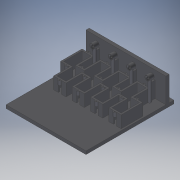
# Autodesk Inventor part: Costas
Saved by Autodesk Inventor 2018 (Build 220112000, 112)
## iProperties
Created: 2017-06-04
Part Number: Costas
Material: Genérico
Document SubType Name: Modeling
Designer: Vitor
Density: 1 g/cm^3
Appearance: Padrão
Author: Vitor
Autodesk Inventor part; units mm, degrees
ref_plane "YZ Plane" through (0, 0, 0) normal (1, 0, 0) x (0, 1, 0)
ref_plane "XZ Plane" through (0, 0, 0) normal (0, 1, 0) x (-1, 0, 0)
ref_plane "XY Plane" through (0, 0, 0) normal (0, 0, 1) x (1, 0, 0)
sketch "Esboço1" plane through (0, 0, 0) normal (0, 0, 1) x (1, 0, 0)
  line L0 (0, 0) -> (100, 0)
  line L1 (100, 0) -> (100, -100)
  line L2 (100, -100) -> (0, -100)
  line L3 (0, -100) -> (0, 0)
  dimension "d0" = 100
  dimension "d1" = 100
  constraints: 8 end point, 2 parallel, 1 horizontal, 1 perpendicular
  measures "d0" distance of L1.end L2.end
  measures "d1" distance of L0.end L1.end
extrude "Extrusão1" add sketch "Esboço1" along normal blind 4
sketch "Esboço2" plane through (0, 0, 4) normal (0, 0, 1) x (1, 0, 0)
  line L0 (100, 0) -> (0, 0) projected
  line L1 (0, 0) -> (4, 0)
  line L2 (4, 0) -> (4, -7)
  line L3 (2, -9) -> (2, -32)
  line L4 (4, -32) -> (4, -9)
  line L5 (2, -32) -> (2, -34)
  line L6 (2, -34) -> (4, -34)
  line L7 (4, -32) -> (15.5, -32)
  line L8 (15.5, -32) -> (15.5, -34)
  line L9 (15.5, -32) -> (13.5, -32)
  line L10 (2, -9) -> (2, -7)
  line L11 (2, -7) -> (4, -7)
  line L12 (15.5, -9) -> (4, -9)
  line L13 (15.5, -7) -> (17.5, -7)
  line L14 (17.5, -7) -> (17.5, -9)
  line L15 (15.5, -9) -> (15.5, -29)
  line L16 (15.5, -29) -> (17.5, -29)
  line L17 (17.5, -27) -> (17.5, -9)
  line L18 (15.5, -29) -> (15.5, -27)
  line L19 (15.5, -29) -> (27, -29)
  line L20 (27, -29) -> (25, -29)
  line L21 (27, -27) -> (27, -29)
  line L22 (25, -27) -> (25, -7)
  line L23 (25, -7) -> (27, -7)
  line L24 (27, -9) -> (27, -27)
  line L25 (15.5, -32) -> (15.5, -52)
  line L26 (15.5, -52) -> (27, -52)
  line L27 (27, -52) -> (27, -32)
  line L28 (13.5, -34) -> (13.5, -52)
  line L29 (13.5, -52) -> (13.5, -54)
  line L30 (13.5, -54) -> (15.5, -54)
  line L31 (27, -54) -> (29, -54)
  line L32 (29, -54) -> (29, -52)
  line L33 (29, -52) -> (29, -34)
  line L34 (29, -32) -> (27, -32)
  line L35 (27, -32) -> (27, -34)
  line L36 (27, -32) -> (38.5, -32)
  line L37 (38.5, -32) -> (36.5, -32)
  line L38 (38.5, -34) -> (38.5, -32)
  line L39 (36.5, -34) -> (36.5, -52)
  line L40 (36.5, -52) -> (36.5, -54)
  line L41 (36.5, -54) -> (38.5, -54)
  line L42 (38.5, -52) -> (38.5, -34)
  line L43 (27, -9) -> (38.5, -9)
  line L44 (38.5, -9) -> (38.5, -27)
  line L45 (38.5, -27) -> (38.5, -29)
  line L46 (38.5, -29) -> (40.5, -29)
  line L47 (40.5, -27) -> (40.5, -9)
  line L48 (40.5, -7) -> (38.5, -7)
  line L49 (40.5, -7) -> (40.5, -9)
  line L50 (38.5, -29) -> (50, -29)
  line L51 (50, -29) -> (50, -27)
  line L52 (50, -52) -> (48, -52)
  line L53 (48, -52) -> (38.5, -52)
  line L54 (50, -34) -> (50, -32)
  line L55 (50, -34) -> (50, -52)
  line L56 (50, -32) -> (52, -32)
  line L57 (52, -34) -> (52, -52)
  line L58 (52, -52) -> (52, -54)
  line L59 (50, -54) -> (52, -54)
  line L60 (50, -32) -> (61.5, -32)
  line L61 (61.5, -32) -> (59.5, -32)
  line L62 (50, -27) -> (50, -9)
  line L63 (50, -7) -> (48, -7)
  line L64 (48, -7) -> (48, -9)
  line L65 (48, -9) -> (48, -27)
  line L66 (50, -9) -> (61.5, -9)
  line L67 (61.5, -7) -> (63.5, -7)
  line L68 (63.5, -7) -> (63.5, -9)
  line L69 (61.5, -9) -> (61.5, -27)
  line L70 (61.5, -27) -> (61.5, -29)
  line L71 (61.5, -29) -> (63.5, -29)
  line L72 (63.5, -27) -> (63.5, -9)
  line L73 (61.5, -34) -> (61.5, -32)
  line L74 (59.5, -34) -> (59.5, -52)
  line L75 (59.5, -52) -> (59.5, -54)
  line L76 (59.5, -54) -> (61.5, -54)
  line L77 (61.5, -52) -> (61.5, -34)
  line L78 (61.5, -52) -> (73, -52)
  line L79 (73, -54) -> (75, -54)
  line L80 (75, -54) -> (75, -52)
  line L81 (73, -52) -> (73, -34)
  line L82 (73, -34) -> (73, -32)
  line L83 (73, -32) -> (75, -32)
  line L84 (75, -34) -> (75, -52)
  line L85 (61.5, -29) -> (73, -29)
  line L86 (73, -29) -> (71, -29)
  line L87 (73, -27) -> (73, -29)
  line L88 (71, -27) -> (71, -9)
  line L89 (71, -9) -> (71, -7)
  line L90 (71, -7) -> (73, -7)
  line L91 (73, -9) -> (73, -27)
  line L92 (73, -9) -> (84.5, -9)
  line L93 (84.5, -7) -> (86.5, -7)
  line L94 (86.5, -7) -> (86.5, -9)
  line L95 (84.5, -9) -> (84.5, -27)
  line L96 (84.5, -27) -> (84.5, -29)
  line L97 (84.5, -29) -> (86.5, -29)
  line L98 (86.5, -27) -> (86.5, -9)
  line L99 (73, -32) -> (84.5, -32)
  line L100 (84.5, -32) -> (84.5, -34)
  line L101 (82.5, -34) -> (82.5, -52)
  line L102 (82.5, -52) -> (82.5, -54)
  line L103 (82.5, -54) -> (84.5, -54)
  line L104 (84.5, -52) -> (84.5, -34)
  line L105 (84.5, -52) -> (96, -52)
  line L106 (96, -54) -> (98, -54)
  line L107 (98, -54) -> (98, -52)
  line L108 (84.5, -29) -> (96, -29)
  line L109 (96, -29) -> (96, -52)
  line L110 (98, -52) -> (98, -29)
  line L111 (98, -29) -> (98, -27)
  line L112 (96, -27) -> (98, -27)
  arc A0 (11.75, -7) -> (7.75, -7) centre (9.75, -7) ccw
  arc A1 (23.25, -27) -> (19.25, -27) centre (21.25, -27) ccw
  arc A2 (19.25, -54) -> (23.25, -54) centre (21.25, -54) ccw
  arc A3 (30.75, -34) -> (34.75, -34) centre (32.75, -34) ccw
  arc A4 (34.75, -7) -> (30.75, -7) centre (32.75, -7) ccw
  arc A5 (46.25, -27) -> (42.25, -27) centre (44.25, -27) ccw
  arc A6 (57.75, -7) -> (53.75, -7) centre (55.75, -7) ccw
  arc A7 (69.25, -27) -> (65.25, -27) centre (67.25, -27) ccw
  arc A8 (80.75, -7) -> (76.75, -7) centre (78.75, -7) ccw
  arc A9 (88.25, -54) -> (92.25, -54) centre (90.25, -54) ccw
  arc A10 (76.75, -34) -> (80.75, -34) centre (78.75, -34) ccw
  arc A11 (65.25, -54) -> (69.25, -54) centre (67.25, -54) ccw
  arc A12 (53.75, -34) -> (57.75, -34) centre (55.75, -34) ccw
  arc A13 (42.25, -54) -> (46.25, -54) centre (44.25, -54) ccw
  line L113 (4, -7) -> (7.75, -7)
  line L114 (11.75, -7) -> (15.5, -7)
  line L115 (27, -7) -> (30.75, -7)
  line L116 (34.75, -7) -> (38.5, -7)
  line L117 (61.5, -7) -> (57.75, -7)
  line L118 (53.75, -7) -> (50, -7)
  line L119 (25, -27) -> (23.25, -27)
  line L120 (19.25, -27) -> (17.5, -27)
  line L121 (84.5, -7) -> (80.75, -7)
  line L122 (76.75, -7) -> (73, -7)
  line L123 (96, -54) -> (92.25, -54)
  line L124 (88.25, -54) -> (84.5, -54)
  line L125 (73, -54) -> (69.25, -54)
  line L126 (65.25, -54) -> (61.5, -54)
  line L127 (38.5, -54) -> (42.25, -54)
  line L128 (46.25, -54) -> (50, -54)
  line L129 (15.5, -54) -> (19.25, -54)
  line L130 (23.25, -54) -> (27, -54)
  line L131 (4, -34) -> (6.75, -34)
  line L132 (11.75, -34) -> (13.5, -34)
  line L133 (36.5, -34) -> (34.75, -34)
  line L134 (30.75, -34) -> (29, -34)
  line L135 (48, -27) -> (46.25, -27)
  line L136 (42.25, -27) -> (40.5, -27)
  line L137 (59.5, -34) -> (57.75, -34)
  line L138 (53.75, -34) -> (52, -34)
  line L139 (63.5, -27) -> (65.25, -27)
  line L140 (69.25, -27) -> (71, -27)
  line L141 (82.5, -34) -> (80.75, -34)
  line L142 (76.75, -34) -> (75, -34)
  line L143 (96, -27) -> (93.25, -27)
  line L144 (88.25, -27) -> (86.5, -27)
  line L145 (92.25, -27) -> (93.25, -27)
  line L146 (6.75, -34) -> (7.75, -34)
  arc A14 (92.25, -27) -> (88.25, -27) centre (90.25, -27) ccw
  arc A15 (7.75, -34) -> (11.75, -34) centre (9.75, -34) ccw
  dimension "d4" = 4
  constraints: 292 end point, 65 point on line, 37 perpendicular, 32 point on circle, 16 centre point, 9 horizontal, 8 vertical, 3 parallel
  measures "d4" distance of L0.end L1.end
extrude "Extrusão3" add sketch "Esboço2" along normal blind 15
sketch "Esboço3" plane through (0, 0, 19) normal (0, 0, 1) x (1, 0, 0)
  line L0 (15.5, -9) -> (4, -9) projected
  line L1 (9.75, -9) -> (9.75, -6.7)
  line L2 (9.75, -6.7) -> (32.75, -6.7)
  line L3 (32.75, -6.7) -> (55.75, -6.7)
  line L4 (55.75, -6.7) -> (78.75, -6.7)
  line L5 (78.75, -6.7) -> (78.75, -34.3)
  line L6 (78.75, -34.3) -> (55.75, -34.3)
  line L7 (55.75, -34.3) -> (32.75, -34.3)
  line L8 (32.75, -34.3) -> (9.75, -34.3)
  line L9 (15.5, -29) -> (27, -29) projected
  line L10 (21.25, -29) -> (21.25, -26.7)
  line L11 (21.25, -26.7) -> (44.25, -26.7)
  line L12 (44.25, -26.7) -> (67.25, -26.7)
  line L13 (67.25, -26.7) -> (90.25, -26.7)
  line L14 (90.25, -26.7) -> (90.25, -54.3)
  line L15 (90.25, -54.3) -> (67.25, -54.3)
  line L16 (88.25, -54) -> (82.5, -54) projected
  line L17 (90.25, -54.3) -> (113.25, -54.3) construction
  line L18 (67.25, -54.3) -> (44.25, -54.3)
  line L19 (44.25, -54.3) -> (21.25, -54.3)
  circle A0 centre (21.25, -54.3) radius 0.75
  circle A1 centre (44.25, -54.3) radius 0.75
  circle A2 centre (67.25, -54.3) radius 0.75
  circle A3 centre (90.25, -54.3) radius 0.75
  circle A4 centre (90.25, -26.7) radius 0.75
  circle A5 centre (78.75, -34.3) radius 0.75
  circle A6 centre (67.25, -26.7) radius 0.75
  circle A7 centre (55.75, -34.3) radius 0.75
  circle A8 centre (44.25, -26.7) radius 0.75
  circle A9 centre (32.75, -34.3) radius 0.75
  circle A10 centre (21.25, -26.7) radius 0.75
  circle A11 centre (9.75, -34.3) radius 0.75
  circle A12 centre (9.75, -6.7) radius 0.75
  circle A13 centre (32.75, -6.7) radius 0.75
  circle A14 centre (55.75, -6.7) radius 0.75
  circle A15 centre (78.75, -6.7) radius 0.75
  point P0 (0, 0)
  dimension "d88" = 2.3
  dimension "d89" = 23
  dimension "d90" = 23
  dimension "d91" = 23
  dimension "d92" = 27.6
  dimension "d93" = 23
  dimension "d94" = 23
  dimension "d95" = 23
  dimension "d96" = 2.3
  dimension "d97" = 23
  dimension "d98" = 23
  dimension "d99" = 23
  dimension "d100" = 27.6
  dimension "d101" = 23
  dimension "d102" = 180
  dimension "d103" = 23
  dimension "d104" = 23
  dimension "d105" = 1.5
  dimension "d106" = 1.5
  dimension "d107" = 1.5
  dimension "d108" = 1.5
  dimension "d109" = 1.5
  dimension "d110" = 1.5
  dimension "d111" = 1.5
  dimension "d112" = 1.5
  dimension "d113" = 1.5
  dimension "d114" = 1.5
  dimension "d115" = 1.5
  dimension "d116" = 1.5
  dimension "d117" = 1.5
  dimension "d118" = 1.5
  dimension "d119" = 1.5
  dimension "d120" = 1.5
  constraints: 34 end point, 16 centre point, 16 coincident, 8 point on line, 5 perpendicular, 2 midpoint, 2 vertical, 1 collinear, 1 horizontal, 1 parallel
  measures "d88" distance of L1.start L1.end
  measures "d89" distance of L1.end L2.end
  measures "d90" distance of L2.end L3.end
  measures "d91" distance of L3.end L4.end
  measures "d92" distance of L4.end L5.end
  measures "d93" distance of L5.end L6.end
  measures "d94" distance of L6.end L7.end
  measures "d95" distance of L7.end L8.end
  measures "d96" distance of L10.start L10.end
  measures "d97" distance of L10.end L11.end
  measures "d98" distance of L11.end L12.end
  measures "d99" distance of L12.end L13.end
  measures "d100" distance of L13.end L14.end
  measures "d101" distance of L14.end L15.end
  measures "d102" angle of L15 L17
  measures "d103" distance of L15.end L18.end
  measures "d104" distance of L18.end L19.end
  measures "d105" diameter of A0
  measures "d106" diameter of A1
  measures "d107" diameter of A2
  measures "d108" diameter of A3
  measures "d109" diameter of A4
  measures "d110" diameter of A5
  measures "d111" diameter of A6
  measures "d112" diameter of A7
  measures "d113" diameter of A8
  measures "d114" diameter of A9
  measures "d115" diameter of A10
  measures "d116" diameter of A11
  measures "d117" diameter of A12
  measures "d118" diameter of A13
  measures "d119" diameter of A14
  measures "d120" diameter of A15
extrude "Extrusão4" cut sketch "Esboço3" against normal blind 10
sketch "Esboço4" plane through (0, 0, 4) normal (0, 0, 1) x (1, 0, 0)
  line L0 (17.5, -7) -> (11.75, -7) projected
  circle A0 centre (17.5, -7) radius 2
  circle A1 centre (40.6139, -7) radius 2
  line L1 (63.5, -27) -> (63.5, -7) projected
  circle A2 centre (63.5, -7) radius 2
  line L2 (86.5, -7) -> (80.75, -7) projected
  circle A3 centre (86.5, -7) radius 2
  point P0 (0, 0)
  dimension "d123" = 4
  dimension "d124" = 4
  dimension "d125" = 4
  dimension "d126" = 4
  constraints: 4 centre point
  measures "d123" diameter of A0
  measures "d124" diameter of A1
  measures "d125" diameter of A2
  measures "d126" diameter of A3
extrude "Extrusão5" add sketch "Esboço4" along normal blind 25
sketch "Esboço5" plane through (86.5, -7, 29) normal (0, 0, 1) x (1, 0, 0)
  line L0 (0, 0) -> (-1, 0)
  line L1 (-1, 0) -> (-1, 1)
  line L2 (-1, 1) -> (1, 1)
  line L3 (1, 1) -> (1, 0)
  line L4 (1, 0) -> (0, 0)
  circle A0 centre (-23, 0) radius 2 projected
  line L5 (-23, 0) -> (-24, 0)
  line L6 (-24, 0) -> (-24, 1)
  line L7 (-24, 1) -> (-22, 1)
  line L8 (-22, 1) -> (-22, 0)
  line L9 (-22, 0) -> (-23, 0)
  arc A1 (-46, -1.9968) -> (-47.8861, 0) centre (-45.8861, 0) ccw projected
  line L10 (-45.8861, 0) -> (-44.8861, 0)
  line L11 (-44.8861, 0) -> (-44.8861, 1)
  line L12 (-44.8861, 1) -> (-46.8861, 1)
  line L13 (-46.8861, 1) -> (-46.8861, 0)
  line L14 (-46.8861, 0) -> (-45.8861, 0)
  circle A2 centre (-69, 0) radius 2 projected
  line L15 (-69, 0) -> (-70, 0)
  line L16 (-70, 0) -> (-70, 1)
  line L17 (-70, 1) -> (-68, 1)
  line L18 (-68, 1) -> (-68, 0)
  line L19 (-68, 0) -> (-69, 0)
  point P0 (-86.5, 7)
  dimension "d129" = 1
  dimension "d130" = 1
  dimension "d131" = 2
  dimension "d132" = 1
  dimension "d133" = 2
  dimension "d134" = 1
  dimension "d135" = 1
  dimension "d136" = 1
  dimension "d137" = 2
  dimension "d138" = 1
  dimension "d139" = 1
  dimension "d140" = 2
  dimension "d141" = 1
  constraints: 40 end point, 11 perpendicular, 10 point on line, 1 horizontal, 1 vertical
  measures "d129" distance of L0.start L0.end
  measures "d130" distance of L0.end L1.end
  measures "d131" distance of L1.end L2.end
  measures "d132" distance of L5.start L5.end
  measures "d133" distance of L6.end L7.end
  measures "d134" distance of L7.end L8.end
  measures "d135" distance of L10.start L10.end
  measures "d136" distance of L10.end L11.end
  measures "d137" distance of L11.end L12.end
  measures "d138" distance of L15.start L15.end
  measures "d139" distance of L15.end L16.end
  measures "d140" distance of L16.end L17.end
  measures "d141" distance of L17.end L18.end
extrude "Extrusão6" add sketch "Esboço5" along normal blind 2 contours L0 L1 L2 L3 L4 | L5 L6 L7 L8 L9 | L14 L13 L12 L11 L10 | L15 L16 L17 L18 L19
sketch "Esboço6" plane through (62.5, -6, 29) normal (0, 1, 0) x (1, 0, 0)
  line L0 (2, -2) -> (0, -2) projected
  circle A0 centre (1, -2) radius 3
  line L1 (25, -2) -> (23, -2) projected
  circle A1 centre (24, -2) radius 3
  line L2 (-22.8861, -2) -> (-20.8861, -2) projected
  circle A2 centre (-21.8861, -2) radius 3
  line L3 (-46, -2) -> (-44, -2) projected
  circle A3 centre (-45, -2) radius 3
  point P0 (-62.5, 29)
  dimension "d144" = 6
  dimension "d145" = 6
  dimension "d146" = 6
  dimension "d147" = 6
  constraints: 4 centre point, 4 midpoint
  measures "d144" diameter of A0
  measures "d145" diameter of A1
  measures "d146" diameter of A2
  measures "d147" diameter of A3
extrude "Extrusão7" add sketch "Esboço6" along normal blind 2 and the other way blind 1
sketch "Esboço7" plane through (61.5, -7, 29) normal (0, -1, 0) x (1, 0, 0)
  circle A0 centre (-44, 2) radius 3 projected
  circle A1 centre (-44, 2) radius 3
  circle A2 centre (-20.8861, 2) radius 3 projected
  circle A3 centre (-20.8861, 2) radius 3
  circle A4 centre (2, 2) radius 3 projected
  circle A5 centre (2, 2) radius 3
  circle A6 centre (25, 2) radius 3 projected
  circle A7 centre (25, 2) radius 3
  point P0 (-61.5, -29)
  dimension "d152" = 6
  dimension "d153" = 6
  dimension "d154" = 6
  dimension "d155" = 6
  constraints: 4 centre point, 4 coincident
  measures "d152" diameter of A1
  measures "d153" diameter of A3
  measures "d154" diameter of A5
  measures "d155" diameter of A7
extrude "Extrusão8" add sketch "Esboço7" along normal blind 3
sketch "Esboço8" plane through (17.5, -10, 31) normal (0, -1, 0) x (1, 0, 0)
  circle A0 centre (0, 0) radius 3 projected
  circle A1 centre (0, 0) radius 1.5
  circle A2 centre (23.1139, 0) radius 3 projected
  circle A3 centre (23.1139, 0) radius 1.5
  circle A4 centre (46, 0) radius 3 projected
  circle A5 centre (46, 0) radius 1.5
  circle A6 centre (69, 0) radius 3 projected
  circle A7 centre (69, 0) radius 1.5
  point P0 (-17.5, -31)
  dimension "d158" = 3
  dimension "d159" = 3
  dimension "d160" = 3
  dimension "d161" = 3
  constraints: 4 centre point, 4 coincident
  measures "d158" diameter of A1
  measures "d159" diameter of A3
  measures "d160" diameter of A5
  measures "d161" diameter of A7
extrude "Extrusão9" cut sketch "Esboço8" against normal blind 7 contours A1 | A3 | A5 | A7
fillet "Arredondamento1" radius 1 8 edges at (39.1139, -10, 31) (62, -10, 31) (85, -10, 31) (16, -10, 31) (85, -4, 31) (62, -4, 31) (39.1139, -4, 31) (16, -4, 31)
sketch "Esboço9" plane through (2, -34, 4) normal (0, -1, 0) x (1, 0, 0)
  line L0 (5.75, 0) -> (5.75, 15) projected
  line L1 (5.75, 0) -> (5.75, 10)
  line L2 (5.75, 10) -> (9.75, 10)
  line L3 (9.75, 0) -> (9.75, 15) projected
  line L4 (9.75, 10) -> (9.75, 0)
  line L5 (9.75, 0) -> (5.75, 0)
  line L6 (2, 0) -> (13.5, 0) projected
  line L7 (28.75, 0) -> (28.75, 15) projected
  line L8 (28.75, 0) -> (28.75, 10)
  line L9 (28.75, 10) -> (32.75, 10)
  line L10 (32.75, 0) -> (32.75, 15) projected
  line L11 (32.75, 0) -> (28.75, 0)
  line L12 (51.75, 0) -> (55.75, 0) projected
  line L13 (51.75, 0) -> (55.75, 0)
  line L14 (28.75, 10) -> (32.75, 10)
  line L15 (51.75, 0) -> (51.75, 10)
  line L16 (51.75, 10) -> (55.75, 10)
  line L17 (55.75, 0) -> (55.75, 15) projected
  line L18 (55.75, 10) -> (55.75, 0)
  line L19 (55.75, 0) -> (51.75, 0)
  line L20 (74.75, 0) -> (74.75, 15) projected
  line L21 (74.75, 0) -> (74.75, 10)
  line L22 (74.75, 10) -> (78.75, 10)
  line L23 (78.75, 0) -> (78.75, 15) projected
  line L24 (78.75, 10) -> (78.75, 0)
  line L25 (98, 0) -> (-2, 0) projected
  line L26 (78.75, 0) -> (74.75, 0)
  line L27 (55.75, 10) -> (51.75, 10)
  line L28 (55.75, 0) -> (51.75, 0)
  line L29 (32.75, 10) -> (28.75, 10)
  line L30 (32.75, 10) -> (32.75, 0)
  line L31 (28.75, 0) -> (32.75, 0) projected
  line L32 (32.75, 0) -> (28.75, 0)
  line L33 (5.75, 10) -> (9.75, 10)
  line L34 (11.5, 0) -> (9.75, 0) projected
  line L35 (5.75, 0) -> (9.75, 0)
  point P0 (-2, -4)
  dimension "d165" = 10
  dimension "d166" = 4
  dimension "d167" = 10
  dimension "d168" = 10
  dimension "d169" = 10
  constraints: 48 end point, 10 collinear, 8 point on line, 3 horizontal, 3 perpendicular, 2 other
  measures "d165" distance of L0.start L1.end
  measures "d166" distance of L1.end L2.end
  measures "d167" distance of L7.start L8.end
  measures "d168" distance of L12.start L15.end
  measures "d169" distance of L20.start L21.end
extrude "Extrusão10" cut sketch "Esboço9" along normal blind 7 and the other way blind 3.5
sketch "Esboço10" plane through (13.5, -54, 4) normal (0, -1, 0) x (1, 0, 0)
  line L0 (5.75, 0) -> (5.75, 15) projected
  line L1 (5.75, 0) -> (5.75, 10)
  line L2 (5.75, 10) -> (9.75, 10)
  line L3 (9.75, 0) -> (9.75, 15) projected
  line L4 (9.75, 0) -> (9.75, 10)
  line L5 (9.75, 0) -> (5.75, 0)
  line L6 (2, 0) -> (13.5, 0) projected
  line L7 (28.75, 0) -> (28.75, 15) projected
  line L8 (28.75, 0) -> (28.75, 10)
  line L9 (28.75, 10) -> (32.75, 10)
  line L10 (32.75, 0) -> (32.75, 15) projected
  line L11 (32.75, 10) -> (32.75, 0)
  line L12 (32.75, 0) -> (28.75, 0)
  line L13 (51.75, 0) -> (51.75, 15) projected
  line L14 (51.75, 0) -> (51.75, 10)
  line L15 (51.75, 10) -> (55.75, 10)
  line L16 (55.75, 0) -> (55.75, 15) projected
  line L17 (55.75, 10) -> (55.75, 0)
  line L18 (55.75, 0) -> (51.75, 0)
  line L19 (48, 0) -> (59.5, 0) projected
  line L20 (74.75, 0) -> (78.75, 0) projected
  line L21 (74.75, 0) -> (74.75, 10)
  line L22 (74.75, 0) -> (74.75, 15) projected
  line L23 (74.75, 10) -> (78.75, 10)
  line L24 (78.75, 0) -> (78.75, 15) projected
  line L25 (78.75, 10) -> (78.75, 0)
  line L26 (78.75, 0) -> (74.75, 0)
  point P0 (-13.5, -4)
  dimension "d174" = 10
  dimension "d175" = 10
  dimension "d176" = 10
  dimension "d177" = 10
  constraints: 32 end point, 11 point on line, 6 collinear, 3 perpendicular
  measures "d174" distance of L0.start L1.end
  measures "d175" distance of L7.start L8.end
  measures "d176" distance of L13.start L14.end
  measures "d177" distance of L20.start L21.end
extrude "Extrusão11" cut sketch "Esboço10" against normal blind 7 and the other way blind 3.5
sketch "Esboço11" plane through (0, 0, 0) normal (0, 1, 0) x (1, 0, 0)
  line L0 (0, 0) -> (100, 0)
  line L1 (100, 0) -> (100, -4)
  line L2 (100, -4) -> (0, -4)
  line L3 (0, -4) -> (0, 0)
  constraints: 8 end point, 2 parallel, 1 horizontal, 1 perpendicular
extrude "Extrusão12" add sketch "Esboço11" along normal blind 10
sketch "Esboço12" plane through (0, 0, 4) normal (0, 0, 1) x (1, 0, 0)
  line L0 (100, -100) -> (100, 10) projected
  line L1 (0, 0) -> (100, 0)
  line L2 (100, 0) -> (100, 4)
  line L3 (100, 4) -> (0, 4)
  line L4 (0, 4) -> (0, 0)
  line L5 (80.75, -7) -> (84.5, -7) projected
  line L6 (84.5, -7) -> (84.5, 0)
  line L7 (86.5, -7) -> (86.5, 0)
  line L8 (86.5, -9) -> (86.5, -27) projected
  line L9 (86.5, -7) -> (84.5, -7)
  line L10 (57.75, -7) -> (61.5, -7) projected
  line L11 (61.5, -7) -> (61.5, 0)
  line L12 (63.5, -7) -> (63.5, 0)
  line L13 (63.5, -9) -> (63.5, -27) projected
  line L14 (63.5, -7) -> (61.5, -7)
  line L15 (34.75, -7) -> (38.6139, -7) projected
  line L16 (38.6139, -7) -> (38.6139, 0)
  line L17 (40.5, -7) -> (40.5, 0)
  line L18 (11.75, -7) -> (15.5, -7) projected
  line L19 (15.5, -7) -> (15.5, 0)
  line L20 (17.5, -7) -> (17.5, 0)
  line L21 (17.5, -9) -> (17.5, -27) projected
  line L22 (15.5, -7) -> (17.5, -7)
  line L23 (38.6139, -7) -> (40.5, -7)
  line L24 (61.5, -7) -> (63.5, -7)
  dimension "d184" = 4
  constraints: 32 end point, 6 vertical, 5 collinear, 4 point on line, 3 perpendicular, 1 horizontal, 1 parallel, 11 other
  measures "d184" distance of L2.end L2.start
extrude "Extrusão13" add sketch "Esboço12" along normal blind 20
sketch "Esboço13" plane through (0, 0, 24) normal (0, 0, 1) x (1, 0, 0)
  line L0 (0, 4) -> (0, 0) projected
  line L1 (0, 0) -> (100, 0)
  line L2 (100, 0) -> (100, 4)
  line L3 (100, 4) -> (0, 4)
  line L4 (0, 4) -> (0, 0)
  dimension "d187" = 100
  dimension "d188" = 4
  constraints: 8 end point, 2 parallel, 1 horizontal, 1 perpendicular
  measures "d187" distance of L3.end L2.end
  measures "d188" distance of L2.end L1.end
extrude "Extrusão14" add sketch "Esboço13" along normal blind 11
sketch "Esboço14" plane through (17.5, 0, 4) normal (0, -1, 0) x (1, 0, 0)
  point P0 (-17.5, -4)
